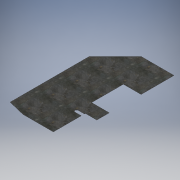
# Autodesk Inventor part: Gearbox-Side Cover Part 1
Saved by Autodesk Inventor 2018 (Build 220112000, 112)
## iProperties
Created: 2018-08-07
Part Number: Gearbox-Side Cover Part 1
Material: Steel
Document SubType Name: Modeling
Designer: P301319
Density: 7.85 g/cm^3
Appearance: Plate
Sheet Metal Rule: Default
Author: P301319
Autodesk Inventor part; units mm, degrees
ref_plane "YZ Plane" through (0, 0, 0) normal (1, 0, 0) x (0, 1, 0)
ref_plane "XZ Plane" through (0, 0, 0) normal (0, 1, 0) x (-1, 0, 0)
ref_plane "XY Plane" through (0, 0, 0) normal (0, 0, 1) x (1, 0, 0)
sketch "Sketch1" plane through (0, 0, 0) normal (0, 0, 1) x (1, 0, 0)
  line L0 (0, 0) -> (223, 0)
  line L1 (0, 0) -> (-123, 30)
  line L2 (0, 0) -> (236.9147, 0) construction
  line L3 (-123, 609.0812) -> (-123, 30)
  line L4 (67.9188, 800) -> (307, 800)
  line L5 (307, 800) -> (307, 560)
  line L6 (307, 560) -> (177, 560)
  line L7 (223, 235) -> (307, 235)
  line L8 (307, 325) -> (307, 235)
  line L9 (178, 203.5) -> (223, 203.5)
  line L10 (178, 228.5) -> (223, 228.5)
  arc A0 (178, 228.5) -> (178, 203.5) centre (178, 216) ccw
  line L11 (223, 0) -> (223, 203.5)
  line L12 (223, 228.5) -> (223, 235)
  line L13 (177, 560) -> (177, 325)
  line L14 (177, 325) -> (307, 325)
  line L15 (67.9188, 800) -> (-123, 609.0812)
  line L16 (67.9188, 800) -> (337.9188, 800) construction
  dimension "d0" = 223
  dimension "d3" = 123
  dimension "d6" = 800
  dimension "d7" = 240
  dimension "d8" = 130
  dimension "d11" = 235
  dimension "d14" = 25
  dimension "d16" = 216
  dimension "d18" = 45
  dimension "d19" = 430
  dimension "d22" = 130
  dimension "d23" = 235
  dimension "d25" = 30
  dimension "d26" = 270
  dimension "d27" = 135
  constraints: 36 end point, 7 horizontal, 4 perpendicular, 4 vertical, 2 point on circle, 2 tangent, 1 centre point, 1 equal length, 1 parallel, 1 vertical alignment
  measures "d0" distance of L0.start L0.end
  measures "d3" distance from line of L0.start L3
  measures "d6" distance between parallel lines of L0 L4
  measures "d7" distance of L4.end L5.end
  measures "d8" distance of L5.end L6.end
  measures "d11" distance of L0.end L7.start
  measures "d14" distance between parallel lines of L9 L10
  measures "d16" vertical distance of L0.start A0.centre
  measures "d18" distance of L9.start L9.end
  measures "d19" distance between parallel lines of L3 L5
  measures "d22" distance of L13.end L8.start
  measures "d23" distance of L6.end L13.end
  measures "d25" vertical distance of L0.start L1.end
  measures "d26" distance of L3.start L4.start
  measures "d27" angle of L15 L16
extrude "Extrusion1" add sketch "Sketch1" along normal blind 1.6
equation "\"d22\" = d8"
equation "\"BendRadius\" = Thickness"
equation "\"BendReliefWidth\" = Thickness"
equation "\"BendReliefDepth\" = 0.5 * Thickness"
equation "\"CornerReliefSize\" = 4 * Thickness"
equation "\"MinimumRemnant\" = 2 * Thickness"
equation "\"TransitionRadius\" = BendRadius"
equation "\"JacobiRadiusSize\" = Thickness"
equation "\"GapSize\" = Thickness"
equation "\"Thickness\" = 0.5"
body "Solid1"
